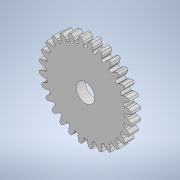
# Autodesk Inventor part: m1歯数28ギア3td6
Saved by Autodesk Inventor 2020.2 (Build 242310000, 310)
## iProperties
Created: 2020-02-29
Part Number: m1歯数28ギア3td6
Material: 一般
Document SubType Name: Modeling
Designer: aoyam
Density: 1 g/cm^3
Appearance: 既定
Author: aoyam
Autodesk Inventor part; units mm, degrees
ref_plane "YZ Plane" through (0, 0, 0) normal (1, 0, 0) x (0, 1, 0)
ref_plane "XZ Plane" through (0, 0, 0) normal (0, 1, 0) x (-1, 0, 0)
ref_plane "XY Plane" through (0, 0, 0) normal (0, 0, 1) x (1, 0, 0)
sketch "スケッチ1" plane through (0, 0, 0) normal (0, 0, 1) x (1, 0, 0)
  arc A0 (-1.8959, 17.685) -> (-1.9245, 17.5003) centre (-0.6833, 17.4027) ccw
  arc A1 (-1.7118, 18.2609) -> (-1.8959, 17.685) centre (1.4401, 16.9362) ccw
  arc A2 (-1.1505, 19.298) -> (-1.7118, 18.2609) centre (3.727, 15.9875) ccw
  arc A3 (-3.0081, 17.5003) -> (-3.0367, 17.685) centre (-4.2493, 17.4027) ccw
  arc A4 (-3.0367, 17.685) -> (-3.2208, 18.2609) centre (-6.3727, 16.9362) ccw
  arc A5 (-3.2208, 18.2609) -> (-3.7821, 19.298) centre (-8.6596, 15.9875) ccw
  arc A6 (-1.9412, 17.095) -> (-2.9914, 17.095) centre (-2.4663, 4.3558) ccw
  arc A7 (-3.7821, 19.298) -> (-4.5084, 19.2161) centre (-2.4663, 4.3558) ccw
  line L0 (-1.9412, 17.095) -> (-1.9245, 17.5003)
  line L1 (-2.9914, 17.095) -> (-3.0081, 17.5003)
  line L2 (-5.813, 16.6587) -> (-5.9194, 17.0502)
  arc A8 (-5.9194, 17.0502) -> (-5.9884, 17.2239) centre (-7.1078, 16.6788) ccw
  arc A9 (-5.9884, 17.2239) -> (-6.296, 17.7444) centre (-9.0742, 15.7515) ccw
  arc A10 (-6.296, 17.7444) -> (-7.074, 18.6306) centre (-11.0926, 14.3177) ccw
  arc A11 (-7.074, 18.6306) -> (-7.764, 18.3891) centre (-2.4663, 4.3558) ccw
  arc A12 (-4.7891, 16.8924) -> (-5.813, 16.6587) centre (-2.4663, 4.3558) ccw
  line L3 (-4.7891, 16.8924) -> (-4.863, 17.2913)
  arc A13 (-4.8762, 17.4777) -> (-4.863, 17.2913) centre (-3.6312, 17.4723) ccw
  arc A14 (-4.8249, 18.0802) -> (-4.8762, 17.4777) centre (-1.4572, 17.49) ccw
  arc A15 (-4.5084, 19.2161) -> (-4.8249, 18.0802) centre (0.9834, 17.074) ccw
  line L4 (-8.4667, 15.6056) -> (-8.6576, 15.9635)
  arc A16 (-8.6576, 15.9635) -> (-8.7635, 16.1175) centre (-9.7335, 15.3371) ccw
  arc A17 (-8.7635, 16.1175) -> (-9.1793, 16.5566) centre (-11.4443, 13.9954) ccw
  arc A18 (-9.1793, 16.5566) -> (-10.1349, 17.2473) centre (-13.0931, 12.1484) ccw
  arc A19 (-10.1349, 17.2473) -> (-10.7539, 16.8584) centre (-2.4663, 4.3558) ccw
  arc A20 (-7.5205, 16.0612) -> (-8.4667, 15.6056) centre (-2.4663, 4.3558) ccw
  line L5 (-7.5205, 16.0612) -> (-7.6813, 16.4337)
  arc A21 (-7.7357, 16.6125) -> (-7.6813, 16.4337) centre (-6.5207, 16.8843) ccw
  arc A22 (-7.8198, 17.2113) -> (-7.7357, 16.6125) centre (-4.4052, 17.3853) ccw
  arc A23 (-7.764, 18.3891) -> (-7.8198, 17.2113) centre (-1.9331, 17.5227) ccw
  line L6 (-10.8196, 13.9883) -> (-11.0854, 14.2948)
  arc A24 (-11.0854, 14.2948) -> (-11.2229, 14.4213) centre (-11.9949, 13.4446) ccw
  arc A25 (-11.2229, 14.4213) -> (-11.7259, 14.7569) centre (-13.3642, 11.7559) ccw
  arc A26 (-11.7259, 14.7569) -> (-12.8113, 15.2177) centre (-14.5606, 9.5883) ccw
  arc A27 (-12.8113, 15.2177) -> (-13.3282, 14.7008) centre (-2.4663, 4.3558) ccw
  arc A28 (-9.9985, 14.6431) -> (-10.8196, 13.9883) centre (-2.4663, 4.3558) ccw
  line L7 (-9.9985, 14.6431) -> (-10.2382, 14.9704)
  arc A29 (-10.331, 15.1326) -> (-10.2382, 14.9704) centre (-9.2069, 15.668) ccw
  arc A30 (-10.5461, 15.6977) -> (-10.331, 15.1326) centre (-7.2559, 16.6271) ccw
  arc A31 (-10.7539, 16.8584) -> (-10.5461, 15.6977) centre (-4.8764, 17.3113) ccw
  line L8 (-12.7536, 11.888) -> (-13.0809, 12.1277)
  arc A32 (-13.0809, 12.1277) -> (-13.2431, 12.2205) centre (-13.7784, 11.0964) ccw
  arc A33 (-13.2431, 12.2205) -> (-13.8082, 12.4357) centre (-14.7376, 9.1454) ccw
  arc A34 (-13.8082, 12.4357) -> (-14.9689, 12.6434) centre (-15.4218, 6.7659) ccw
  arc A35 (-14.9689, 12.6434) -> (-15.3578, 12.0245) centre (-2.4663, 4.3558) ccw
  arc A36 (-12.0988, 12.7091) -> (-12.7536, 11.888) centre (-2.4663, 4.3558) ccw
  line L9 (-12.0988, 12.7091) -> (-12.4053, 12.9749)
  arc A37 (-12.5318, 13.1124) -> (-12.4053, 12.9749) centre (-11.5551, 13.8844) ccw
  arc A38 (-12.8674, 13.6154) -> (-12.5318, 13.1124) centre (-9.8664, 15.2537) ccw
  arc A39 (-13.3282, 14.7008) -> (-12.8674, 13.6154) centre (-7.6988, 16.4501) ccw
  line L10 (-14.1717, 9.41) -> (-14.5442, 9.5709)
  arc A40 (-14.5442, 9.5709) -> (-14.723, 9.6252) centre (-14.9948, 8.4102) ccw
  arc A41 (-14.723, 9.6252) -> (-15.3218, 9.7093) centre (-15.4957, 6.2947) ccw
  arc A42 (-15.3218, 9.7093) -> (-16.4996, 9.6535) centre (-15.6332, 3.8226) ccw
  arc A43 (-16.4996, 9.6535) -> (-16.741, 8.9635) centre (-2.4663, 4.3558) ccw
  arc A44 (-13.7161, 10.3562) -> (-14.1717, 9.41) centre (-2.4663, 4.3558) ccw
  line L11 (-13.7161, 10.3562) -> (-14.074, 10.5471)
  arc A45 (-14.228, 10.653) -> (-14.074, 10.5471) centre (-13.4475, 11.623) ccw
  arc A46 (-14.667, 11.0688) -> (-14.228, 10.653) centre (-12.1059, 13.3338) ccw
  arc A47 (-15.3578, 12.0245) -> (-14.667, 11.0688) centre (-10.2589, 14.9826) ccw
  line L12 (-15.0029, 6.6786) -> (-15.4018, 6.7525)
  arc A48 (-15.4018, 6.7525) -> (-15.5882, 6.7657) centre (-15.5828, 5.5207) ccw
  arc A49 (-15.5882, 6.7657) -> (-16.1907, 6.7144) centre (-15.6005, 3.3467) ccw
  arc A50 (-16.1907, 6.7144) -> (-17.3266, 6.3979) centre (-15.1845, 0.9061) ccw
  arc A51 (-17.3266, 6.3979) -> (-17.4085, 5.6716) centre (-2.4663, 4.3558) ccw
  arc A52 (-14.7692, 7.7025) -> (-15.0029, 6.6786) centre (-2.4663, 4.3558) ccw
  line L13 (-14.7692, 7.7025) -> (-15.1607, 7.809)
  arc A53 (-15.3344, 7.8779) -> (-15.1607, 7.809) centre (-14.7893, 8.9973) ccw
  arc A54 (-15.8549, 8.1855) -> (-15.3344, 7.8779) centre (-13.862, 10.9637) ccw
  arc A55 (-16.741, 8.9635) -> (-15.8549, 8.1855) centre (-12.4282, 12.9821) ccw
  line L14 (-15.2055, 3.8307) -> (-15.6108, 3.814)
  arc A56 (-15.6108, 3.814) -> (-15.7955, 3.7854) centre (-15.5132, 2.5728) ccw
  arc A57 (-15.7955, 3.7854) -> (-16.3714, 3.6013) centre (-15.0467, 0.4494) ccw
  arc A58 (-16.3714, 3.6013) -> (-17.4085, 3.04) centre (-14.098, -1.8375) ccw
  arc A59 (-17.4085, 3.04) -> (-17.3266, 2.3137) centre (-2.4663, 4.3558) ccw
  arc A60 (-15.2055, 4.8809) -> (-15.2055, 3.8307) centre (-2.4663, 4.3558) ccw
  line L15 (-15.2055, 4.8809) -> (-15.6108, 4.8976)
  arc A61 (-15.7955, 4.9262) -> (-15.6108, 4.8976) centre (-15.5132, 6.1388) ccw
  arc A62 (-16.3714, 5.1103) -> (-15.7955, 4.9262) centre (-15.0467, 8.2622) ccw
  arc A63 (-17.4085, 5.6716) -> (-16.3714, 5.1103) centre (-14.098, 10.5491) ccw
  line L16 (-14.7692, 1.0091) -> (-15.1607, 0.9026)
  arc A64 (-15.1607, 0.9026) -> (-15.3344, 0.8337) centre (-14.7893, -0.2857) ccw
  arc A65 (-15.3344, 0.8337) -> (-15.8549, 0.5261) centre (-13.862, -2.2521) ccw
  arc A66 (-15.8549, 0.5261) -> (-16.741, -0.2519) centre (-12.4282, -4.2705) ccw
  arc A67 (-16.741, -0.2519) -> (-16.4996, -0.9419) centre (-2.4663, 4.3558) ccw
  arc A68 (-15.0029, 2.033) -> (-14.7692, 1.0091) centre (-2.4663, 4.3558) ccw
  line L17 (-15.0029, 2.033) -> (-15.4018, 1.9591)
  arc A69 (-15.5882, 1.9459) -> (-15.4018, 1.9591) centre (-15.5828, 3.1909) ccw
  arc A70 (-16.1907, 1.9972) -> (-15.5882, 1.9459) centre (-15.6005, 5.3649) ccw
  arc A71 (-17.3266, 2.3137) -> (-16.1907, 1.9972) centre (-15.1845, 7.8055) ccw
  line L18 (-13.7161, -1.6446) -> (-14.074, -1.8355)
  arc A72 (-14.074, -1.8355) -> (-14.228, -1.9414) centre (-13.4475, -2.9114) ccw
  arc A73 (-14.228, -1.9414) -> (-14.667, -2.3572) centre (-12.1059, -4.6222) ccw
  arc A74 (-14.667, -2.3572) -> (-15.3578, -3.3129) centre (-10.2589, -6.271) ccw
  arc A75 (-15.3578, -3.3129) -> (-14.9689, -3.9318) centre (-2.4663, 4.3558) ccw
  arc A76 (-14.1717, -0.6984) -> (-13.7161, -1.6446) centre (-2.4663, 4.3558) ccw
  line L19 (-14.1717, -0.6984) -> (-14.5442, -0.8593)
  arc A77 (-14.723, -0.9136) -> (-14.5442, -0.8593) centre (-14.9948, 0.3014) ccw
  arc A78 (-15.3218, -0.9977) -> (-14.723, -0.9136) centre (-15.4957, 2.4169) ccw
  arc A79 (-16.4996, -0.9419) -> (-15.3218, -0.9977) centre (-15.6332, 4.889) ccw
  line L20 (-12.0988, -3.9975) -> (-12.4053, -4.2633)
  arc A80 (-12.4053, -4.2633) -> (-12.5318, -4.4008) centre (-11.5551, -5.1728) ccw
  arc A81 (-12.5318, -4.4008) -> (-12.8674, -4.9038) centre (-9.8664, -6.5421) ccw
  arc A82 (-12.8674, -4.9038) -> (-13.3282, -5.9892) centre (-7.6988, -7.7385) ccw
  arc A83 (-13.3282, -5.9892) -> (-12.8113, -6.5061) centre (-2.4663, 4.3558) ccw
  arc A84 (-12.7536, -3.1764) -> (-12.0988, -3.9975) centre (-2.4663, 4.3558) ccw
  line L21 (-12.7536, -3.1764) -> (-13.0809, -3.4161)
  arc A85 (-13.2431, -3.5089) -> (-13.0809, -3.4161) centre (-13.7784, -2.3848) ccw
  arc A86 (-13.8082, -3.724) -> (-13.2431, -3.5089) centre (-14.7376, -0.4338) ccw
  arc A87 (-14.9689, -3.9318) -> (-13.8082, -3.724) centre (-15.4218, 1.9457) ccw
  line L22 (-9.9985, -5.9315) -> (-10.2382, -6.2588)
  arc A88 (-10.2382, -6.2588) -> (-10.331, -6.421) centre (-9.2069, -6.9563) ccw
  arc A89 (-10.331, -6.421) -> (-10.5461, -6.9861) centre (-7.2559, -7.9155) ccw
  arc A90 (-10.5461, -6.9861) -> (-10.7539, -8.1468) centre (-4.8764, -8.5997) ccw
  arc A91 (-10.7539, -8.1468) -> (-10.1349, -8.5357) centre (-2.4663, 4.3558) ccw
  arc A92 (-10.8196, -5.2767) -> (-9.9985, -5.9315) centre (-2.4663, 4.3558) ccw
  line L23 (-10.8196, -5.2767) -> (-11.0854, -5.5832)
  arc A93 (-11.2229, -5.7097) -> (-11.0854, -5.5832) centre (-11.9949, -4.733) ccw
  arc A94 (-11.7259, -6.0453) -> (-11.2229, -5.7097) centre (-13.3642, -3.0443) ccw
  arc A95 (-12.8113, -6.5061) -> (-11.7259, -6.0453) centre (-14.5606, -0.8767) ccw
  line L24 (-7.5205, -7.3496) -> (-7.6813, -7.7221)
  arc A96 (-7.6813, -7.7221) -> (-7.7357, -7.9009) centre (-6.5207, -8.1727) ccw
  arc A97 (-7.7357, -7.9009) -> (-7.8198, -8.4997) centre (-4.4052, -8.6737) ccw
  arc A98 (-7.8198, -8.4997) -> (-7.764, -9.6775) centre (-1.9331, -8.8111) ccw
  arc A99 (-7.764, -9.6775) -> (-7.074, -9.919) centre (-2.4663, 4.3558) ccw
  arc A100 (-8.4667, -6.894) -> (-7.5205, -7.3496) centre (-2.4663, 4.3558) ccw
  line L25 (-8.4667, -6.894) -> (-8.6576, -7.2519)
  arc A101 (-8.7635, -7.4059) -> (-8.6576, -7.2519) centre (-9.7335, -6.6255) ccw
  arc A102 (-9.1793, -7.845) -> (-8.7635, -7.4059) centre (-11.4443, -5.2838) ccw
  arc A103 (-10.1349, -8.5357) -> (-9.1793, -7.845) centre (-13.0931, -3.4368) ccw
  line L26 (-4.7891, -8.1808) -> (-4.863, -8.5797)
  arc A104 (-4.863, -8.5797) -> (-4.8762, -8.7661) centre (-3.6312, -8.7607) ccw
  arc A105 (-4.8762, -8.7661) -> (-4.8249, -9.3686) centre (-1.4572, -8.7784) ccw
  arc A106 (-4.8249, -9.3686) -> (-4.5084, -10.5045) centre (0.9834, -8.3624) ccw
  arc A107 (-4.5084, -10.5045) -> (-3.7821, -10.5864) centre (-2.4663, 4.3558) ccw
  arc A108 (-5.813, -7.9471) -> (-4.7891, -8.1808) centre (-2.4663, 4.3558) ccw
  line L27 (-5.813, -7.9471) -> (-5.9194, -8.3386)
  arc A109 (-5.9884, -8.5123) -> (-5.9194, -8.3386) centre (-7.1078, -7.9672) ccw
  arc A110 (-6.296, -9.0328) -> (-5.9884, -8.5123) centre (-9.0742, -7.0399) ccw
  arc A111 (-7.074, -9.919) -> (-6.296, -9.0328) centre (-11.0926, -5.6061) ccw
  line L28 (-1.9412, -8.3834) -> (-1.9245, -8.7887)
  arc A112 (-1.9245, -8.7887) -> (-1.8959, -8.9734) centre (-0.6833, -8.6911) ccw
  arc A113 (-1.8959, -8.9734) -> (-1.7118, -9.5493) centre (1.4401, -8.2246) ccw
  arc A114 (-1.7118, -9.5493) -> (-1.1505, -10.5864) centre (3.727, -7.2759) ccw
  arc A115 (-1.1505, -10.5864) -> (-0.4241, -10.5045) centre (-2.4663, 4.3558) ccw
  arc A116 (-2.9914, -8.3834) -> (-1.9412, -8.3834) centre (-2.4663, 4.3558) ccw
  line L29 (-2.9914, -8.3834) -> (-3.0081, -8.7887)
  arc A117 (-3.0367, -8.9734) -> (-3.0081, -8.7887) centre (-4.2493, -8.6911) ccw
  arc A118 (-3.2208, -9.5493) -> (-3.0367, -8.9734) centre (-6.3727, -8.2246) ccw
  arc A119 (-3.7821, -10.5864) -> (-3.2208, -9.5493) centre (-8.6596, -7.2759) ccw
  line L30 (0.8804, -7.9471) -> (0.9869, -8.3386)
  arc A120 (0.9869, -8.3386) -> (1.0558, -8.5123) centre (2.1752, -7.9672) ccw
  arc A121 (1.0558, -8.5123) -> (1.3634, -9.0328) centre (4.1416, -7.0399) ccw
  arc A122 (1.3634, -9.0328) -> (2.1415, -9.919) centre (6.16, -5.6061) ccw
  arc A123 (2.1415, -9.919) -> (2.8314, -9.6775) centre (-2.4663, 4.3558) ccw
  arc A124 (-0.1435, -8.1808) -> (0.8804, -7.9471) centre (-2.4663, 4.3558) ccw
  line L31 (-0.1435, -8.1808) -> (-0.0696, -8.5797)
  arc A125 (-0.0564, -8.7661) -> (-0.0696, -8.5797) centre (-1.3014, -8.7607) ccw
  arc A126 (-0.1077, -9.3686) -> (-0.0564, -8.7661) centre (-3.4754, -8.7784) ccw
  arc A127 (-0.4241, -10.5045) -> (-0.1077, -9.3686) centre (-5.916, -8.3624) ccw
  line L32 (3.5341, -6.894) -> (3.7251, -7.2519)
  arc A128 (3.7251, -7.2519) -> (3.8309, -7.4059) centre (4.801, -6.6255) ccw
  arc A129 (3.8309, -7.4059) -> (4.2467, -7.845) centre (6.5117, -5.2838) ccw
  arc A130 (4.2467, -7.845) -> (5.2024, -8.5357) centre (8.1605, -3.4368) ccw
  arc A131 (5.2024, -8.5357) -> (5.8213, -8.1468) centre (-2.4663, 4.3558) ccw
  arc A132 (2.5879, -7.3496) -> (3.5341, -6.894) centre (-2.4663, 4.3558) ccw
  line L33 (2.5879, -7.3496) -> (2.7488, -7.7221)
  arc A133 (2.8031, -7.9009) -> (2.7488, -7.7221) centre (1.5881, -8.1727) ccw
  arc A134 (2.8872, -8.4997) -> (2.8031, -7.9009) centre (-0.5274, -8.6737) ccw
  arc A135 (2.8314, -9.6775) -> (2.8872, -8.4997) centre (-2.9995, -8.8111) ccw
  line L34 (5.887, -5.2767) -> (6.1528, -5.5832)
  arc A136 (6.1528, -5.5832) -> (6.2903, -5.7097) centre (7.0623, -4.733) ccw
  arc A137 (6.2903, -5.7097) -> (6.7933, -6.0453) centre (8.4316, -3.0443) ccw
  arc A138 (6.7933, -6.0453) -> (7.8787, -6.5061) centre (9.6281, -0.8767) ccw
  arc A139 (7.8787, -6.5061) -> (8.3956, -5.9892) centre (-2.4663, 4.3558) ccw
  arc A140 (5.0659, -5.9315) -> (5.887, -5.2767) centre (-2.4663, 4.3558) ccw
  line L35 (5.0659, -5.9315) -> (5.3056, -6.2588)
  arc A141 (5.3984, -6.421) -> (5.3056, -6.2588) centre (4.2743, -6.9563) ccw
  arc A142 (5.6136, -6.9861) -> (5.3984, -6.421) centre (2.3233, -7.9155) ccw
  arc A143 (5.8213, -8.1468) -> (5.6136, -6.9861) centre (-0.0562, -8.5997) ccw
  line L36 (7.821, -3.1764) -> (8.1483, -3.4161)
  arc A144 (8.1483, -3.4161) -> (8.3105, -3.5089) centre (8.8459, -2.3848) ccw
  arc A145 (8.3105, -3.5089) -> (8.8756, -3.724) centre (9.805, -0.4338) ccw
  arc A146 (8.8756, -3.724) -> (10.0364, -3.9318) centre (10.4892, 1.9457) ccw
  arc A147 (10.0364, -3.9318) -> (10.4252, -3.3129) centre (-2.4663, 4.3558) ccw
  arc A148 (7.1662, -3.9975) -> (7.821, -3.1764) centre (-2.4663, 4.3558) ccw
  line L37 (7.1662, -3.9975) -> (7.4727, -4.2633)
  arc A149 (7.5993, -4.4008) -> (7.4727, -4.2633) centre (6.6225, -5.1728) ccw
  arc A150 (7.9348, -4.9038) -> (7.5993, -4.4008) centre (4.9338, -6.5421) ccw
  arc A151 (8.3956, -5.9892) -> (7.9348, -4.9038) centre (2.7662, -7.7385) ccw
  line L38 (9.2391, -0.6984) -> (9.6116, -0.8593)
  arc A152 (9.6116, -0.8593) -> (9.7904, -0.9136) centre (10.0622, 0.3014) ccw
  arc A153 (9.7904, -0.9136) -> (10.3892, -0.9977) centre (10.5632, 2.4169) ccw
  arc A154 (10.3892, -0.9977) -> (11.567, -0.9419) centre (10.7006, 4.889) ccw
  arc A155 (11.567, -0.9419) -> (11.8085, -0.2519) centre (-2.4663, 4.3558) ccw
  arc A156 (8.7835, -1.6446) -> (9.2391, -0.6984) centre (-2.4663, 4.3558) ccw
  line L39 (8.7835, -1.6446) -> (9.1414, -1.8355)
  arc A157 (9.2954, -1.9414) -> (9.1414, -1.8355) centre (8.515, -2.9114) ccw
  arc A158 (9.7345, -2.3572) -> (9.2954, -1.9414) centre (7.1733, -4.6222) ccw
  arc A159 (10.4252, -3.3129) -> (9.7345, -2.3572) centre (5.3263, -6.271) ccw
  line L40 (10.0703, 2.033) -> (10.4692, 1.9591)
  arc A160 (10.4692, 1.9591) -> (10.6556, 1.9459) centre (10.6503, 3.1909) ccw
  arc A161 (10.6556, 1.9459) -> (11.2581, 1.9972) centre (10.6679, 5.3649) ccw
  arc A162 (11.2581, 1.9972) -> (12.394, 2.3137) centre (10.2519, 7.8055) ccw
  arc A163 (12.394, 2.3137) -> (12.4759, 3.04) centre (-2.4663, 4.3558) ccw
  arc A164 (9.8366, 1.0091) -> (10.0703, 2.033) centre (-2.4663, 4.3558) ccw
  line L41 (9.8366, 1.0091) -> (10.2281, 0.9026)
  arc A165 (10.4018, 0.8337) -> (10.2281, 0.9026) centre (9.8568, -0.2857) ccw
  arc A166 (10.9223, 0.5261) -> (10.4018, 0.8337) centre (8.9294, -2.2521) ccw
  arc A167 (11.8085, -0.2519) -> (10.9223, 0.5261) centre (7.4956, -4.2705) ccw
  line L42 (10.2729, 4.8809) -> (10.6782, 4.8976)
  arc A168 (10.6782, 4.8976) -> (10.8629, 4.9262) centre (10.5806, 6.1388) ccw
  arc A169 (10.8629, 4.9262) -> (11.4389, 5.1103) centre (10.1141, 8.2622) ccw
  arc A170 (11.4389, 5.1103) -> (12.4759, 5.6716) centre (9.1654, 10.5491) ccw
  arc A171 (12.4759, 5.6716) -> (12.394, 6.3979) centre (-2.4663, 4.3558) ccw
  arc A172 (10.2729, 3.8307) -> (10.2729, 4.8809) centre (-2.4663, 4.3558) ccw
  line L43 (10.2729, 3.8307) -> (10.6782, 3.814)
  arc A173 (10.8629, 3.7854) -> (10.6782, 3.814) centre (10.5806, 2.5728) ccw
  arc A174 (11.4389, 3.6013) -> (10.8629, 3.7854) centre (10.1141, 0.4494) ccw
  arc A175 (12.4759, 3.04) -> (11.4389, 3.6013) centre (9.1654, -1.8375) ccw
  line L44 (9.8366, 7.7025) -> (10.2281, 7.809)
  arc A176 (10.2281, 7.809) -> (10.4018, 7.8779) centre (9.8568, 8.9973) ccw
  arc A177 (10.4018, 7.8779) -> (10.9223, 8.1855) centre (8.9294, 10.9637) ccw
  arc A178 (10.9223, 8.1855) -> (11.8085, 8.9635) centre (7.4956, 12.9821) ccw
  arc A179 (11.8085, 8.9635) -> (11.567, 9.6535) centre (-2.4663, 4.3558) ccw
  arc A180 (10.0703, 6.6786) -> (9.8366, 7.7025) centre (-2.4663, 4.3558) ccw
  line L45 (10.0703, 6.6786) -> (10.4692, 6.7525)
  arc A181 (10.6556, 6.7657) -> (10.4692, 6.7525) centre (10.6503, 5.5207) ccw
  arc A182 (11.2581, 6.7144) -> (10.6556, 6.7657) centre (10.6679, 3.3467) ccw
  arc A183 (12.394, 6.3979) -> (11.2581, 6.7144) centre (10.2519, 0.9061) ccw
  line L46 (8.7835, 10.3562) -> (9.1414, 10.5471)
  arc A184 (9.1414, 10.5471) -> (9.2954, 10.653) centre (8.515, 11.623) ccw
  arc A185 (9.2954, 10.653) -> (9.7345, 11.0688) centre (7.1733, 13.3338) ccw
  arc A186 (9.7345, 11.0688) -> (10.4252, 12.0245) centre (5.3263, 14.9826) ccw
  arc A187 (10.4252, 12.0245) -> (10.0364, 12.6434) centre (-2.4663, 4.3558) ccw
  arc A188 (9.2391, 9.41) -> (8.7835, 10.3562) centre (-2.4663, 4.3558) ccw
  line L47 (9.2391, 9.41) -> (9.6116, 9.5709)
  arc A189 (9.7904, 9.6252) -> (9.6116, 9.5709) centre (10.0622, 8.4102) ccw
  arc A190 (10.3892, 9.7093) -> (9.7904, 9.6252) centre (10.5632, 6.2947) ccw
  arc A191 (11.567, 9.6535) -> (10.3892, 9.7093) centre (10.7006, 3.8226) ccw
  line L48 (7.1662, 12.7091) -> (7.4727, 12.9749)
  arc A192 (7.4727, 12.9749) -> (7.5993, 13.1124) centre (6.6225, 13.8844) ccw
  arc A193 (7.5993, 13.1124) -> (7.9348, 13.6154) centre (4.9338, 15.2537) ccw
  arc A194 (7.9348, 13.6154) -> (8.3956, 14.7008) centre (2.7662, 16.4501) ccw
  arc A195 (8.3956, 14.7008) -> (7.8787, 15.2177) centre (-2.4663, 4.3558) ccw
  arc A196 (7.821, 11.888) -> (7.1662, 12.7091) centre (-2.4663, 4.3558) ccw
  line L49 (7.821, 11.888) -> (8.1483, 12.1277)
  arc A197 (8.3105, 12.2205) -> (8.1483, 12.1277) centre (8.8459, 11.0964) ccw
  arc A198 (8.8756, 12.4357) -> (8.3105, 12.2205) centre (9.805, 9.1454) ccw
  arc A199 (10.0364, 12.6434) -> (8.8756, 12.4357) centre (10.4892, 6.7659) ccw
  line L50 (5.0659, 14.6431) -> (5.3056, 14.9704)
  arc A200 (5.3056, 14.9704) -> (5.3984, 15.1326) centre (4.2743, 15.668) ccw
  arc A201 (5.3984, 15.1326) -> (5.6136, 15.6977) centre (2.3233, 16.6271) ccw
  arc A202 (5.6136, 15.6977) -> (5.8213, 16.8584) centre (-0.0562, 17.3113) ccw
  arc A203 (5.8213, 16.8584) -> (5.2024, 17.2473) centre (-2.4663, 4.3558) ccw
  arc A204 (5.887, 13.9883) -> (5.0659, 14.6431) centre (-2.4663, 4.3558) ccw
  line L51 (5.887, 13.9883) -> (6.1528, 14.2948)
  arc A205 (6.2903, 14.4213) -> (6.1528, 14.2948) centre (7.0623, 13.4446) ccw
  arc A206 (6.7933, 14.7569) -> (6.2903, 14.4213) centre (8.4316, 11.7559) ccw
  arc A207 (7.8787, 15.2177) -> (6.7933, 14.7569) centre (9.6281, 9.5883) ccw
  line L52 (2.5879, 16.0612) -> (2.7488, 16.4337)
  arc A208 (2.7488, 16.4337) -> (2.8031, 16.6125) centre (1.5881, 16.8843) ccw
  arc A209 (2.8031, 16.6125) -> (2.8872, 17.2113) centre (-0.5274, 17.3853) ccw
  arc A210 (2.8872, 17.2113) -> (2.8314, 18.3891) centre (-2.9995, 17.5227) ccw
  arc A211 (2.8314, 18.3891) -> (2.1415, 18.6306) centre (-2.4663, 4.3558) ccw
  arc A212 (3.5341, 15.6056) -> (2.5879, 16.0612) centre (-2.4663, 4.3558) ccw
  line L53 (3.5341, 15.6056) -> (3.7251, 15.9635)
  arc A213 (3.8309, 16.1175) -> (3.7251, 15.9635) centre (4.801, 15.3371) ccw
  arc A214 (4.2467, 16.5566) -> (3.8309, 16.1175) centre (6.5117, 13.9954) ccw
  arc A215 (5.2024, 17.2473) -> (4.2467, 16.5566) centre (8.1605, 12.1484) ccw
  line L54 (-0.1435, 16.8924) -> (-0.0696, 17.2913)
  arc A216 (-0.0696, 17.2913) -> (-0.0564, 17.4777) centre (-1.3014, 17.4723) ccw
  arc A217 (-0.0564, 17.4777) -> (-0.1077, 18.0802) centre (-3.4754, 17.49) ccw
  arc A218 (-0.1077, 18.0802) -> (-0.4241, 19.2161) centre (-5.916, 17.074) ccw
  arc A219 (-0.4241, 19.2161) -> (-1.1505, 19.298) centre (-2.4663, 4.3558) ccw
  arc A220 (0.8804, 16.6587) -> (-0.1435, 16.8924) centre (-2.4663, 4.3558) ccw
  line L55 (0.8804, 16.6587) -> (0.9869, 17.0502)
  arc A221 (1.0558, 17.2239) -> (0.9869, 17.0502) centre (2.1752, 16.6788) ccw
  arc A222 (1.3634, 17.7444) -> (1.0558, 17.2239) centre (4.1416, 15.7515) ccw
  arc A223 (2.1415, 18.6306) -> (1.3634, 17.7444) centre (6.16, 14.3177) ccw
  circle A224 centre (-2.4663, 4.3558) radius 3
  point P0 (0, 0)
  point P1 (-1.9412, 17.095)
  point P2 (-2.9914, 17.095)
  point P3 (-3.0367, 17.685)
  point P4 (-3.2208, 18.2609)
  point P5 (-3.7821, 19.298)
  point P6 (-4.5084, 19.2161)
  point P7 (-4.8249, 18.0802)
  point P8 (-4.8762, 17.4777)
  point P9 (-4.863, 17.2913)
  point P10 (-5.9884, 17.2239)
  point P11 (-6.296, 17.7444)
  point P12 (-7.074, 18.6306)
  point P13 (-7.764, 18.3891)
  point P14 (-7.8198, 17.2113)
  point P15 (-7.7357, 16.6125)
  point P16 (-8.6576, 15.9635)
  point P17 (-9.1793, 16.5566)
  point P18 (-10.1349, 17.2473)
  point P19 (-10.7539, 16.8584)
  point P20 (-10.5461, 15.6977)
  point P21 (-10.331, 15.1326)
  point P22 (-10.2382, 14.9704)
  point P23 (-9.9985, 14.6431)
  point P24 (-10.8196, 13.9883)
  point P25 (-11.2229, 14.4213)
  point P26 (-11.7259, 14.7569)
  point P27 (-12.8113, 15.2177)
  point P28 (-13.3282, 14.7008)
  point P29 (-12.8674, 13.6154)
  point P30 (-12.5318, 13.1124)
  point P31 (-12.4053, 12.9749)
  point P32 (-12.0988, 12.7091)
  point P33 (-12.7536, 11.888)
  point P34 (-13.2431, 12.2205)
  point P35 (-13.8082, 12.4357)
  point P36 (-14.9689, 12.6434)
  point P37 (-15.3578, 12.0245)
  point P38 (-14.667, 11.0688)
  point P39 (-14.228, 10.653)
  point P40 (-14.074, 10.5471)
  point P41 (-13.7161, 10.3562)
  point P42 (-14.1717, 9.41)
  point P43 (-14.5442, 9.5709)
  point P44 (-14.723, 9.6252)
  point P45 (-15.3218, 9.7093)
  point P46 (-16.4996, 9.6535)
  point P47 (-16.741, 8.9635)
  point P48 (-15.8549, 8.1855)
  point P49 (-15.3344, 7.8779)
  point P50 (-14.7692, 7.7025)
  point P51 (-15.0029, 6.6786)
  point P52 (-15.4018, 6.7525)
  point P53 (-15.5882, 6.7657)
  point P54 (-16.1907, 6.7144)
  point P55 (-17.3266, 6.3979)
  point P56 (-17.4085, 5.6716)
  point P57 (-16.3714, 5.1103)
  point P58 (-15.7955, 4.9262)
  point P59 (-15.6108, 4.8976)
  point P60 (-15.7955, 3.7854)
  point P61 (-16.3714, 3.6013)
  point P62 (-17.4085, 3.04)
  point P63 (-17.3266, 2.3137)
  point P64 (-16.1907, 1.9972)
  point P65 (-15.5882, 1.9459)
  point P66 (-15.4018, 1.9591)
  point P67 (-15.0029, 2.033)
  point P68 (-14.7692, 1.0091)
  point P69 (-15.1607, 0.9026)
  point P70 (-15.3344, 0.8337)
  point P71 (-15.8549, 0.5261)
  point P72 (-16.741, -0.2519)
  point P73 (-16.4996, -0.9419)
  point P74 (-15.3218, -0.9977)
  point P75 (-14.723, -0.9136)
  point P76 (-14.5442, -0.8593)
  point P77 (-14.228, -1.9414)
  point P78 (-14.667, -2.3572)
  point P79 (-15.3578, -3.3129)
  point P80 (-14.9689, -3.9318)
  point P81 (-13.8082, -3.724)
  point P82 (-13.2431, -3.5089)
  point P83 (-13.0809, -3.4161)
  point P84 (-12.5318, -4.4008)
  point P85 (-12.8674, -4.9038)
  point P86 (-13.3282, -5.9892)
  point P87 (-12.8113, -6.5061)
  point P88 (-11.7259, -6.0453)
  point P89 (-11.2229, -5.7097)
  point P90 (-10.2382, -6.2588)
  point P91 (-10.331, -6.421)
  point P92 (-10.5461, -6.9861)
  point P93 (-10.7539, -8.1468)
  point P94 (-10.1349, -8.5357)
  point P95 (-9.1793, -7.845)
  point P96 (-8.7635, -7.4059)
  point P97 (-8.6576, -7.2519)
  point P98 (-7.7357, -7.9009)
  point P99 (-7.8198, -8.4997)
  point P100 (-7.764, -9.6775)
  point P101 (-7.074, -9.919)
  point P102 (-6.296, -9.0328)
  point P103 (-5.9884, -8.5123)
  point P104 (-5.9194, -8.3386)
  point P105 (-5.813, -7.9471)
  point P106 (-4.7891, -8.1808)
  point P107 (-4.863, -8.5797)
  point P108 (-4.8762, -8.7661)
  point P109 (-4.8249, -9.3686)
  point P110 (-4.5084, -10.5045)
  point P111 (-3.7821, -10.5864)
  point P112 (-3.2208, -9.5493)
  point P113 (-3.0367, -8.9734)
  point P114 (-3.0081, -8.7887)
  point P115 (-2.9914, -8.3834)
  point P116 (-1.8959, -8.9734)
  point P117 (-1.7118, -9.5493)
  point P118 (-1.1505, -10.5864)
  point P119 (-0.4241, -10.5045)
  point P120 (-0.1077, -9.3686)
  point P121 (-0.0564, -8.7661)
  point P122 (-0.0696, -8.5797)
  point P123 (-0.1435, -8.1808)
  point P124 (1.0558, -8.5123)
  point P125 (1.3634, -9.0328)
  point P126 (2.1415, -9.919)
  point P127 (2.8314, -9.6775)
  point P128 (2.8872, -8.4997)
  point P129 (2.8031, -7.9009)
  point P130 (2.7488, -7.7221)
  point P131 (2.5879, -7.3496)
  point P132 (3.5341, -6.894)
  point P133 (3.8309, -7.4059)
  point P134 (4.2467, -7.845)
  point P135 (5.2024, -8.5357)
  point P136 (5.8213, -8.1468)
  point P137 (5.6136, -6.9861)
  point P138 (5.3984, -6.421)
  point P139 (5.887, -5.2767)
  point P140 (6.1528, -5.5832)
  point P141 (6.2903, -5.7097)
  point P142 (6.7933, -6.0453)
  point P143 (7.8787, -6.5061)
  point P144 (8.3956, -5.9892)
  point P145 (7.9348, -4.9038)
  point P146 (7.5993, -4.4008)
  point P147 (7.4727, -4.2633)
  point P148 (8.3105, -3.5089)
  point P149 (8.8756, -3.724)
  point P150 (10.0364, -3.9318)
  point P151 (10.4252, -3.3129)
  point P152 (9.7345, -2.3572)
  point P153 (9.2954, -1.9414)
  point P154 (9.7904, -0.9136)
  point P155 (10.3892, -0.9977)
  point P156 (11.567, -0.9419)
  point P157 (11.8085, -0.2519)
  point P158 (10.9223, 0.5261)
  point P159 (10.4018, 0.8337)
  point P160 (10.4692, 1.9591)
  point P161 (10.6556, 1.9459)
  point P162 (11.2581, 1.9972)
  point P163 (12.394, 2.3137)
  point P164 (12.4759, 3.04)
  point P165 (11.4389, 3.6013)
  point P166 (10.8629, 3.7854)
  point P167 (10.8629, 4.9262)
  point P168 (11.4389, 5.1103)
  point P169 (12.4759, 5.6716)
  point P170 (12.394, 6.3979)
  point P171 (11.2581, 6.7144)
  point P172 (10.6556, 6.7657)
  point P173 (10.4692, 6.7525)
  point P174 (10.4018, 7.8779)
  point P175 (10.9223, 8.1855)
  point P176 (11.8085, 8.9635)
  point P177 (11.567, 9.6535)
  point P178 (10.3892, 9.7093)
  point P179 (9.7904, 9.6252)
  point P180 (9.2954, 10.653)
  point P181 (9.7345, 11.0688)
  point P182 (10.4252, 12.0245)
  point P183 (10.0364, 12.6434)
  point P184 (8.8756, 12.4357)
  point P185 (8.3105, 12.2205)
  point P186 (7.1662, 12.7091)
  point P187 (7.4727, 12.9749)
  point P188 (7.5993, 13.1124)
  point P189 (7.9348, 13.6154)
  point P190 (8.3956, 14.7008)
  point P191 (7.8787, 15.2177)
  point P192 (6.7933, 14.7569)
  point P193 (6.2903, 14.4213)
  point P194 (5.887, 13.9883)
  point P195 (5.0659, 14.6431)
  point P196 (5.3056, 14.9704)
  point P197 (5.3984, 15.1326)
  point P198 (5.6136, 15.6977)
  point P199 (5.8213, 16.8584)
  dimension "d2" = 360
  dimension "d6" = 6
  constraints: 448 point on circle, 225 centre point, 112 end point, 3 coincident, 1063 other
  measures "d6" diameter of A224
extrude "押し出し1" add sketch "スケッチ1" along normal blind 3
